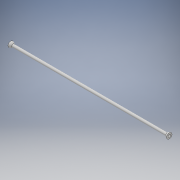
# Autodesk Inventor part: 滑桿
Saved by Autodesk Inventor 2017 (Build 210142000, 142)
## iProperties
Part Number: 滑桿
Material: 一般
Document SubType Name: Modeling
Designer: Brian
Density: 1 g/cm^3
Appearance: 預設
Author: Brian
Autodesk Inventor part; units mm, degrees
ref_plane "YZ Plane" through (0, 0, 0) normal (1, 0, 0) x (0, 1, 0)
ref_plane "XZ Plane" through (0, 0, 0) normal (0, 1, 0) x (-1, 0, 0)
ref_plane "XY Plane" through (0, 0, 0) normal (0, 0, 1) x (1, 0, 0)
sketch "草圖6" plane through (0, 0, 0) normal (0, 0, 1) x (1, 0, 0)
  arc A0 (4.3301, 2.5) -> (5, 0) centre (0, 0) ccw
  arc A1 (285, 0) -> (285.6699, 2.5) centre (290, 0) ccw
  line L0 (0, 0) -> (290, 0)
  line L1 (290, 0) -> (290, 2.5)
  line L2 (285.6699, 2.5) -> (4.3301, 2.5)
  line L3 (0, 2.5) -> (0, 0)
  line L4 (290, 5) -> (290, 2.5)
  line L5 (0, 2.5) -> (0, 5)
  dimension "d20" = 10
  dimension "d21" = 10
  dimension "d22" = 290
  dimension "d23" = 2.5
  dimension "d24" = 2.5
  constraints: 12 end point, 6 point on circle, 2 centre point, 2 coincident, 2 parallel, 2 point on line, 2 vertical, 1 horizontal, 1 perpendicular
  measures "d20" diameter of A1
  measures "d21" diameter of A0
  measures "d22" distance of A1.centre L0.start
  measures "d23" distance of L0.end L1.end
  measures "d24" distance between parallel lines of L2 L0
revolve "迴轉1" add sketch "草圖6" angle 360 about axis through (0, 0, 0) along (1, 0, 0) contours L2 A1 L4 L1 L0 L3 L5 A0
sketch "草圖7" plane through (0, 0, 0) normal (1, 0, 0) x (0, 1, 0)
  circle A0 centre (0, 0) radius 5 projected
  arc A1 (-2.5, 0) -> (2.5, 0) centre (0, 0) ccw
  line L0 (2.5, 0) -> (-2.5, 0)
  dimension "d26" = 5
  dimension "d27" = 5
  constraints: 2 end point, 2 point on circle, 1 centre point, 1 coincident, 1 horizontal
  measures "d26" diameter of A1
  measures "d27" distance of L0.start L0.end
revolve "迴轉2" cut sketch "草圖7" angle 360 about axis through (0, 2.5, 0) along (0, -1, 0) contours L0 A1
sketch "草圖8" plane through (290, 0, 0) normal (1, 0, 0) x (0, 0, -1)
  arc A0 (0, -2.5) -> (0, 2.5) centre (0, 0) ccw
  line L0 (0, 2.5) -> (0, -2.5)
  dimension "d29" = 5
  dimension "d30" = 5
  constraints: 2 end point, 2 point on circle, 1 centre point, 1 coincident, 1 vertical
  measures "d29" diameter of A0
  measures "d30" distance of L0.start L0.end
revolve "迴轉3" cut sketch "草圖8" angle 360 about axis through (290, 2.5, 0) along (0, -1, 0)
